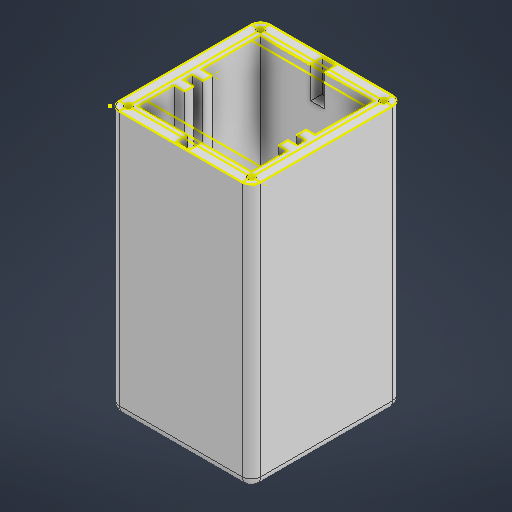
# Autodesk Inventor part: CajaNodoReceptor
Saved by Autodesk Inventor 2027.1 (Build 311270010, 270A)
## iProperties
Created: 2026-09-09
Part Number: CajaNodoReceptor
Material: Genérico
Document SubType Name: Sheet Metal
Designer: marco
Density: 1 g/cm^3
Sheet Metal Rule: Por defecto_mm
Appearance: Valor por defecto
Author: marco
Autodesk Inventor part; units mm, degrees
ref_plane "YZ Plane" through (0, 0, 0) normal (1, 0, 0) x (0, 1, 0)
ref_plane "XZ Plane" through (0, 0, 0) normal (0, 1, 0) x (-1, 0, 0)
ref_plane "XY Plane" through (0, 0, 0) normal (0, 0, 1) x (1, 0, 0)
sketch "Boceto1" plane through (0, 0, 0) normal (0, 1, 0) x (-1, 0, 0)
  line L0 (0, 0) -> (-31, 0)
  line L1 (-31, 0) -> (-31, -33)
  line L2 (-31, -33) -> (0, -33)
  line L3 (0, -33) -> (0, 0)
  line L4 (0, -33) -> (0, -30)
  line L5 (0, -30) -> (0, -15)
  line L6 (0, -15) -> (0, -13)
  line L7 (0, -13) -> (0, -3)
  line L8 (0, -3) -> (0, 0)
  line L9 (0, -30) -> (-31, -30)
  line L10 (0, -15) -> (-31, -15)
  line L11 (0, -13) -> (-31, -13)
  line L12 (0, -3) -> (-31, -3)
  line L13 (0, -33) -> (-3, -33)
  line L14 (0, -33) -> (-3, -33)
  line L15 (-3, -33) -> (-3, 0)
  line L16 (-31, -33) -> (-28, -33)
  line L17 (-28, -33) -> (-28, 0)
  line L18 (-3, -15) -> (-3, -17)
  line L19 (-3, -17) -> (-5.3627, -17)
  line L20 (-5.3627, -17) -> (-5.3627, -15)
  line L21 (-5.3627, -13) -> (-5.3627, -11)
  line L22 (-5.3627, -11) -> (-3, -11)
  line L23 (-28, -15) -> (-26, -15)
  line L24 (-26, -15) -> (-26, -17)
  line L25 (-26, -17) -> (-28, -17)
  line L26 (-26, -13) -> (-26, -11)
  line L27 (-26, -11) -> (-28, -11)
  point P0 (-3, -30)
  point P1 (-28, -30)
  point P2 (-28, -13)
  point P3 (-28, -3)
  point P4 (-3, -3)
  point P5 (-3, -13)
  dimension "d0" = 31
  dimension "d1" = 33
  dimension "d2" = 3
  dimension "d3" = 15
  dimension "d4" = 2
  dimension "d5" = 10
  dimension "d6" = 3
  dimension "d7" = 3
  dimension "d8" = 2
  dimension "d9" = 2
  dimension "d10" = 2
  dimension "d11" = 2
  dimension "d12" = 2
  constraints: 56 end point, 28 point on line, 13 perpendicular, 2 collinear, 2 parallel, 1 horizontal
  measures "d0" distance of L2.end L1.end
  measures "d1" distance of L1.end L0.end
  measures "d2" distance of L2.end L4.end
  measures "d3" distance of L4.end L5.end
  measures "d4" distance of L5.end L6.end
  measures "d5" distance of L6.end L7.end
  measures "d6" distance of L2.end L13.end
  measures "d7" distance of L1.end L16.end
  measures "d8" distance of L18.start L18.end
  measures "d9" distance of L21.start L21.end
  measures "d10" distance of L23.start L23.end
  measures "d11" distance of L23.end L24.end
  measures "d12" distance of L26.start L26.end
extrude "Extrusión1" add sketch "Boceto1" along normal blind 58 contours L3 L12 L15 L0 | L15 L12 L17 L0 | L3 L11 L15 L12 | L17 L12 L1 L0 | L3 L10 L15 L11 | L17 L11 L1 L12 | L15 L11 L21 L22 | L3 L9 L15 L10 | L27 L26 L11 L17 | L3 L2 L15 L9 | L15 L19 L20 L10 | L11 L17 L10 L1 | L15 L2 L17 L9 | L10 L17 L9 L1 | L10 L24 L25 L17 | L17 L2 L1 L9
sketch "Boceto2" plane through (31, 0, 0) normal (1, 0, 0) x (0, 0, -1)
  line L0 (33, 0) -> (33, 58) projected
  line L1 (0, 0) -> (0, 58) projected
  line L2 (33, 0) -> (0, 0)
  line L3 (0, 0) -> (0, 3)
  line L4 (0, 3) -> (33, 3)
  line L5 (33, 3) -> (33, 0)
  dimension "d15" = 3
  constraints: 8 end point, 2 parallel, 1 horizontal, 1 perpendicular, 1 point on line
  measures "d15" distance of L2.end L3.end
extrude "Extrusión2" add sketch "Boceto2" against normal up to surface (28 mm away)
fillet "Empalme1" radius 2 10 edges at (31, 29, 0) (15.5, 0, 0) (31, 0, -16.5) (31, 29, -33) (15.5, 0, -33) (0, 0, -16.5) (0, 29, 0) (0, 29, -33) (15.5, 3, -3) (15.5, 3, -30)
sketch "Boceto4" plane through (0, 58, 0) normal (0, 1, 0) x (1, 0, 0)
  line L0 (0, 31) -> (2, 31) projected
  circle A0 centre (2, 31) radius 0.75
  line L1 (29, 31) -> (31, 31) projected
  circle A1 centre (29, 31) radius 0.75
  line L2 (2, 0) -> (2, 2) projected
  circle A2 centre (2, 2) radius 0.75
  line L3 (2, 2) -> (29, 2) projected
  circle A3 centre (29, 2) radius 0.75
  line L4 (2, 31) -> (15.5, 31)
  line L5 (29, 31) -> (2, 31) projected
  line L6 (14, 29.5) -> (17, 29.5)
  line L7 (17, 29.5) -> (17, 32.5)
  line L8 (17, 32.5) -> (14, 32.5)
  line L9 (14, 32.5) -> (14, 29.5)
  line L10 (14, 29.5) -> (17, 32.5) construction
  line L11 (17, 29.5) -> (14, 32.5) construction
  line L12 (14, 0.5) -> (17, 0.5)
  line L13 (17, 0.5) -> (17, 3.5)
  line L14 (17, 3.5) -> (14, 3.5)
  line L15 (14, 3.5) -> (14, 0.5)
  line L16 (14, 0.5) -> (17, 3.5) construction
  line L17 (17, 0.5) -> (14, 3.5) construction
  point P0 (0, 0)
  point P1 (15.5, 2)
  dimension "d19" = 1.5
  dimension "d20" = 1.5
  dimension "d21" = 1.5
  dimension "d22" = 1.5
  dimension "d23" = 3
  dimension "d24" = 3
  dimension "d25" = 3
  dimension "d26" = 3
  constraints: 26 end point, 6 midpoint, 4 centre point, 4 parallel, 2 horizontal, 2 perpendicular
  measures "d19" diameter of A0
  measures "d20" diameter of A1
  measures "d21" diameter of A2
  measures "d22" diameter of A3
  measures "d23" distance of L8.end L7.end
  measures "d24" distance of L7.end L6.end
  measures "d25" distance of L14.end L13.end
  measures "d26" distance of L13.end L12.end
extrude "Extrusión3" cut sketch "Boceto4" against normal blind 7
sketch "Boceto5" plane through (0, 58, 0) normal (0, 1, 0) x (1, 0, 0)
  line L0 (3, 15) -> (5.3627, 15) projected
  line L1 (3, 28) -> (28, 28) projected
  line L2 (2, 33) -> (29, 33) projected
  arc A0 (2, 33) -> (0, 31) centre (2, 31) ccw projected
  arc A1 (2, 33) -> (0, 31) centre (2, 31) ccw projected
  arc A2 (2, 33) -> (0, 31) centre (2, 31) ccw projected
  line L3 (5.3627, 13) -> (3, 13) projected
  line L4 (5.3627, 11) -> (5.3627, 13) projected
  line L5 (3, 11) -> (5.3627, 11) projected
  line L6 (3, 3) -> (3, 11) projected
  arc A3 (0, 2) -> (2, 0) centre (2, 2) ccw projected
  circle A4 centre (2, 2) radius 0.75 projected
  circle A5 centre (2, 2) radius 0.75 projected
  circle A6 centre (2, 2) radius 0.75 projected
  circle A7 centre (2, 2) radius 0.75 projected
  circle A8 centre (2, 2) radius 0.75 projected
  line L7 (3, 5) -> (3, 11) projected
  line L8 (3, 11) -> (5.3627, 11) projected
  line L9 (5.3627, 11) -> (5.3627, 13) projected
  line L10 (5.3627, 13) -> (3, 13) projected
  line L11 (5.3627, 11) -> (5.3627, 13) projected
  line L12 (5.3627, 11) -> (5.3627, 13) projected
  line L13 (3, 11) -> (5.3627, 11) projected
  line L14 (3, 11) -> (5.3627, 11) projected
  line L15 (3, 3) -> (3, 5) projected
  line L16 (3, 5) -> (3, 11) projected
  line L17 (3, 3) -> (3, 11) projected
  arc A9 (0, 2) -> (2, 0) centre (2, 2) ccw projected
  arc A10 (0, 2) -> (2, 0) centre (2, 2) ccw projected
  line L18 (5.3627, 13) -> (3, 13) projected
  line L19 (5.3627, 13) -> (3, 13) projected
  line L20 (3, 3) -> (28, 3) projected
  line L21 (14, 3) -> (3, 3) projected
  line L22 (28, 3) -> (17, 3) projected
  line L23 (2, 0) -> (29, 0) projected
  line L24 (14, 3) -> (17, 3) projected
  line L25 (17, 3) -> (17, 0.5) projected
  line L26 (17, 3) -> (17, 0.5) projected
  line L27 (14, 0.5) -> (14, 3) projected
  line L28 (14, 0.5) -> (14, 3) projected
  line L29 (17, 0.5) -> (14, 0.5) projected
  line L30 (17, 0.5) -> (14, 0.5) projected
  line L31 (14, 3) -> (17, 3) projected
  line L32 (28, 3) -> (17, 3) projected
  line L33 (3, 3) -> (28, 3) projected
  line L34 (14, 3) -> (3, 3) projected
  line L35 (14, 3) -> (17, 3) projected
  line L36 (14, 0.5) -> (14, 3) projected
  line L37 (17, 0.5) -> (14, 0.5) projected
  line L38 (17, 3) -> (17, 0.5) projected
  line L39 (17, 3) -> (17, 0.5) projected
  line L40 (17, 3) -> (17, 0.5) projected
  line L41 (14, 0.5) -> (14, 3) projected
  line L42 (14, 0.5) -> (14, 3) projected
  line L43 (17, 0.5) -> (14, 0.5) projected
  line L44 (17, 0.5) -> (14, 0.5) projected
  line L45 (28, 5) -> (3, 5) projected
  line L46 (28, 5) -> (28, 3) projected
  line L47 (3, 3) -> (3, 5) projected
  arc A11 (0, 2) -> (2, 0) centre (2, 2) ccw projected
  line L48 (2, 0) -> (29, 0) projected
  line L49 (29, 0) -> (2, 0) projected
  line L50 (26, 17) -> (26, 15) projected
  line L51 (28, 17) -> (26, 17) projected
  line L52 (28, 30) -> (28, 17) projected
  arc A12 (31, 31) -> (29, 33) centre (29, 31) ccw projected
  line L53 (31, 2) -> (31, 31) projected
  circle A13 centre (29, 31) radius 0.75 projected
  circle A14 centre (29, 31) radius 0.75 projected
  circle A15 centre (29, 31) radius 0.75 projected
  circle A16 centre (29, 31) radius 0.75 projected
  circle A17 centre (29, 31) radius 0.75 projected
  line L54 (31, 31) -> (31, 2) projected
  line L55 (31, 31) -> (31, 2) projected
  line L56 (31, 2) -> (31, 31) projected
  line L57 (26, 17) -> (26, 15) projected
  line L58 (26, 17) -> (26, 15) projected
  line L59 (28, 17) -> (26, 17) projected
  line L60 (28, 17) -> (26, 17) projected
  line L61 (28, 30) -> (28, 28) projected
  line L62 (28, 28) -> (28, 17) projected
  line L63 (28, 30) -> (28, 17) projected
  arc A18 (31, 31) -> (29, 33) centre (29, 31) ccw projected
  arc A19 (31, 31) -> (29, 33) centre (29, 31) ccw projected
  line L64 (28, 11) -> (28, 3) projected
  line L65 (26, 11) -> (28, 11) projected
  line L66 (26, 13) -> (26, 11) projected
  line L67 (28, 13) -> (26, 13) projected
  line L68 (28, 15) -> (28, 13) projected
  line L69 (26, 15) -> (28, 15) projected
  arc A20 (29, 0) -> (31, 2) centre (29, 2) ccw projected
  circle A21 centre (29, 2) radius 0.75 projected
  circle A22 centre (29, 2) radius 0.75 projected
  circle A23 centre (29, 2) radius 0.75 projected
  circle A24 centre (29, 2) radius 0.75 projected
  circle A25 centre (29, 2) radius 0.75 projected
  line L70 (26, 13) -> (26, 11) projected
  line L71 (26, 13) -> (26, 11) projected
  line L72 (28, 15) -> (28, 13) projected
  line L73 (28, 15) -> (28, 13) projected
  line L74 (28, 13) -> (26, 13) projected
  line L75 (28, 13) -> (26, 13) projected
  line L76 (26, 11) -> (28, 11) projected
  line L77 (26, 11) -> (28, 11) projected
  line L78 (28, 5) -> (28, 3) projected
  line L79 (28, 11) -> (28, 3) projected
  line L80 (28, 11) -> (28, 5) projected
  arc A26 (29, 0) -> (31, 2) centre (29, 2) ccw projected
  arc A27 (29, 0) -> (31, 2) centre (29, 2) ccw projected
  line L81 (26, 15) -> (28, 15) projected
  line L82 (26, 15) -> (28, 15) projected
  line L83 (28, 30) -> (3, 30) projected
  line L84 (3, 30) -> (14, 30) projected
  line L85 (28, 30) -> (3, 30) projected
  line L86 (17, 30) -> (28, 30) projected
  line L87 (17, 30) -> (14, 30) projected
  line L88 (2, 33) -> (29, 33) projected
  line L89 (29, 33) -> (2, 33) projected
  line L90 (3, 28) -> (3, 30) projected
  line L91 (3, 17) -> (3, 30) projected
  line L92 (3, 17) -> (3, 28) projected
  line L93 (5.3627, 17) -> (3, 17) projected
  line L94 (5.3627, 17) -> (3, 17) projected
  line L95 (5.3627, 15) -> (5.3627, 17) projected
  line L96 (5.3627, 15) -> (5.3627, 17) projected
  line L97 (3, 15) -> (5.3627, 15) projected
  line L98 (3, 15) -> (5.3627, 15) projected
  line L99 (3, 13) -> (3, 15) projected
  line L100 (3, 13) -> (3, 15) projected
  line L101 (17, 30) -> (14, 30) projected
  line L102 (14, 32.5) -> (17, 32.5) projected
  line L103 (17, 30) -> (14, 30) projected
  line L104 (17, 32.5) -> (17, 30) projected
  line L105 (14, 32.5) -> (17, 32.5) projected
  line L106 (14, 30) -> (14, 32.5) projected
  line L107 (17, 30) -> (28, 30) projected
  line L108 (29, 33) -> (2, 33) projected
  arc A28 (29, 0) -> (31, 2) centre (29, 2) ccw projected
  line L109 (31, 2) -> (31, 31) projected
  arc A29 (31, 31) -> (29, 33) centre (29, 31) ccw projected
  line L110 (29, 33) -> (2, 33) projected
  arc A30 (2, 33) -> (0, 31) centre (2, 31) ccw projected
  line L111 (0, 31) -> (0, 2) projected
  arc A31 (0, 2) -> (2, 0) centre (2, 2) ccw projected
  line L112 (2, 0) -> (29, 0) projected
  circle A32 centre (2, 31) radius 0.75 projected
  circle A33 centre (29, 2) radius 0.75 projected
  circle A34 centre (2, 2) radius 0.75 projected
  circle A35 centre (29, 31) radius 0.75 projected
  line L113 (14, 30) -> (14, 32.5) projected
  line L114 (14, 32.5) -> (17, 32.5) projected
  line L115 (17, 32.5) -> (17, 30) projected
  line L116 (17, 30) -> (28, 30) projected
  line L117 (28, 30) -> (28, 17) projected
  line L118 (28, 17) -> (26, 17) projected
  line L119 (26, 17) -> (26, 15) projected
  line L120 (26, 15) -> (28, 15) projected
  line L121 (28, 15) -> (28, 13) projected
  line L122 (28, 13) -> (26, 13) projected
  line L123 (26, 13) -> (26, 11) projected
  line L124 (26, 11) -> (28, 11) projected
  line L125 (28, 11) -> (28, 3) projected
  line L126 (28, 3) -> (17, 3) projected
  line L127 (17, 3) -> (17, 0.5) projected
  line L128 (17, 0.5) -> (14, 0.5) projected
  line L129 (14, 0.5) -> (14, 3) projected
  line L130 (14, 3) -> (3, 3) projected
  line L131 (3, 3) -> (3, 11) projected
  line L132 (3, 11) -> (5.3627, 11) projected
  line L133 (5.3627, 11) -> (5.3627, 13) projected
  line L134 (5.3627, 13) -> (3, 13) projected
  line L135 (3, 13) -> (3, 15) projected
  line L136 (3, 15) -> (5.3627, 15) projected
  line L137 (5.3627, 15) -> (5.3627, 17) projected
  line L138 (5.3627, 17) -> (3, 17) projected
  line L139 (3, 17) -> (3, 30) projected
  line L140 (3, 30) -> (14, 30) projected
  line L141 (5.3627, 15) -> (5.3627, 17) projected
  line L142 (3, 15) -> (5.3627, 15) projected
  line L143 (3, 13) -> (3, 15) projected
  line L144 (5.3627, 17) -> (3, 17) projected
  circle A36 centre (2, 31) radius 0.75 projected
  circle A37 centre (2, 31) radius 0.75 projected
  circle A38 centre (2, 31) radius 0.75 projected
  arc A39 (2, 33) -> (0, 31) centre (2, 31) ccw projected
  line L145 (14, 32.5) -> (17, 32.5) projected
  line L146 (14, 32.5) -> (17, 32.5) projected
  line L147 (14, 32.5) -> (17, 32.5) projected
  line L148 (3, 28) -> (3, 30) projected
  line L149 (5.3627, 17) -> (3, 17) projected
  line L150 (5.3627, 15) -> (5.3627, 17) projected
  arc A40 (2, 33) -> (0, 31) centre (2, 31) ccw projected
  line L151 (2, 31) -> (2, 33) projected
  line L152 (0, 31) -> (2, 31) projected
  line L153 (28, 30) -> (28, 28) projected
  line L154 (26, 17) -> (26, 15) projected
  line L155 (28, 17) -> (26, 17) projected
  line L156 (26, 15) -> (28, 15) projected
  line L157 (26, 13) -> (26, 11) projected
  line L158 (28, 15) -> (28, 13) projected
  line L159 (28, 13) -> (26, 13) projected
  line L160 (26, 11) -> (28, 11) projected
  line L161 (28, 11) -> (28, 5) projected
  line L162 (29, 0) -> (2, 0) projected
  arc A41 (29, 0) -> (31, 2) centre (29, 2) ccw projected
  line L163 (29, 31) -> (2, 31) projected
  line L164 (2, 31) -> (2, 2) projected
  line L165 (29, 2) -> (29, 31) projected
  line L166 (2, 2) -> (29, 2) projected
  line L167 (31, 2) -> (29, 2) projected
  line L168 (29, 2) -> (29, 0) projected
  line L169 (2, 0) -> (2, 2) projected
  line L170 (2, 2) -> (0, 2) projected
  line L171 (29, 33) -> (29, 31) projected
  line L172 (29, 31) -> (31, 31) projected
  line L173 (0, 31) -> (2, 31) projected
  line L174 (2, 31) -> (2, 33) projected
  line L175 (28, 30) -> (28, 28) projected
  line L176 (28, 30) -> (3, 30) projected
  line L177 (3, 28) -> (3, 30) projected
  line L178 (3, 28) -> (28, 28) projected
  line L179 (3, 3) -> (3, 5) projected
  line L180 (3, 3) -> (28, 3) projected
  line L181 (28, 5) -> (28, 3) projected
  line L182 (28, 5) -> (3, 5) projected
  arc A42 (31, 31) -> (29, 33) centre (29, 31) ccw projected
  line L183 (29, 31) -> (31, 31) projected
  line L184 (29, 33) -> (29, 31) projected
  line L185 (2, 2) -> (29, 2) projected
  line L186 (2, 31) -> (2, 2) projected
  line L187 (29, 31) -> (2, 31) projected
  line L188 (29, 2) -> (29, 31) projected
  line L189 (2, 2) -> (0, 2) projected
  line L190 (0, 2) -> (0, 31) projected
  line L191 (0, 31) -> (2, 31) projected
  line L192 (2, 31) -> (2, 2) projected
  line L193 (29, 31) -> (31, 31) projected
  line L194 (31, 31) -> (31, 2) projected
  line L195 (31, 2) -> (29, 2) projected
  line L196 (29, 2) -> (29, 31) projected
  line L197 (2, 2) -> (0, 2) projected
  line L198 (2, 0) -> (2, 2) projected
  arc A43 (0, 2) -> (2, 0) centre (2, 2) ccw projected
  arc A44 (29, 0) -> (31, 2) centre (29, 2) ccw projected
  line L199 (29, 2) -> (29, 0) projected
  line L200 (31, 2) -> (29, 2) projected
  line L201 (29, 2) -> (29, 0) projected
  line L202 (29, 0) -> (2, 0) projected
  line L203 (2, 0) -> (2, 2) projected
  line L204 (2, 2) -> (29, 2) projected
  line L205 (3, 28) -> (28, 28) projected
  line L206 (3, 17) -> (3, 28) projected
  line L207 (5.3627, 17) -> (3, 17) projected
  line L208 (5.3627, 15) -> (5.3627, 17) projected
  line L209 (3, 15) -> (5.3627, 15) projected
  line L210 (3, 13) -> (3, 15) projected
  line L211 (5.3627, 13) -> (3, 13) projected
  line L212 (5.3627, 11) -> (5.3627, 13) projected
  line L213 (3, 11) -> (5.3627, 11) projected
  line L214 (3, 5) -> (3, 11) projected
  line L215 (28, 5) -> (3, 5) projected
  line L216 (28, 11) -> (28, 5) projected
  line L217 (26, 11) -> (28, 11) projected
  line L218 (26, 13) -> (26, 11) projected
  line L219 (28, 13) -> (26, 13) projected
  line L220 (28, 15) -> (28, 13) projected
  line L221 (26, 15) -> (28, 15) projected
  line L222 (26, 17) -> (26, 15) projected
  line L223 (28, 17) -> (26, 17) projected
  line L224 (28, 28) -> (28, 17) projected
  line L225 (3, 17) -> (3, 28) projected
  circle A45 centre (2, 31) radius 0.75 projected
  circle A46 centre (2, 31) radius 0.75 projected
  line L226 (3, 17) -> (3, 30) projected
  line L227 (17, 32.5) -> (17, 30) projected
  line L228 (17, 32.5) -> (17, 30) projected
  line L229 (17, 32.5) -> (17, 30) projected
  line L230 (17, 32.5) -> (17, 30) projected
  line L231 (14, 30) -> (14, 32.5) projected
  line L232 (14, 30) -> (14, 32.5) projected
  line L233 (14, 30) -> (14, 32.5) projected
  line L234 (14, 30) -> (14, 32.5) projected
  line L235 (3, 30) -> (14, 30) projected
  arc A47 (31, 31) -> (29, 33) centre (29, 31) ccw projected
  line L236 (2, 31) -> (2, 33) projected
  line L237 (2, 33) -> (29, 33) projected
  line L238 (29, 33) -> (29, 31) projected
  line L239 (29, 31) -> (2, 31) projected
  line L240 (28, 28) -> (28, 17) projected
  line L241 (3, 13) -> (3, 15) projected
  point P0 (0, 0)
  constraints: 29 other
equation "\"Radio_pliegue\" = Grosor"
equation "\"Anchura_desahogo_plegado\" = Grosor"
equation "\"Profundidad_desahogo_plegado\" = 0.5 * Grosor"
equation "\"Tamaño_destalonado\" = 4 * Grosor"
equation "\"Remanente_mínimo\" = 2 * Grosor"
equation "\"Radiodetransición\" = Radio_pliegue"
equation "\"Tamaño_de_radio_de_Jacobi\" = Radio_pliegue"
equation "\"TamañoSeparación\" = Grosor"
equation "\"Grosor\" = 0.5"
